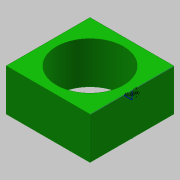
# Autodesk Inventor part: B2-Y
Saved by Autodesk Inventor 2018.1 (Build 221171000, 171)
## iProperties
Created: 2018-06-22
Part Number: B2-Y
Material: Všeobecné
Document SubType Name: Modeling
Designer: PS
Density: 1 g/cm^3
Appearance: Výchozí
Author: PS
Autodesk Inventor part; units mm, degrees
ref_plane "YZ Plane" through (0, 0, 0) normal (1, 0, 0) x (0, 1, 0)
ref_plane "XZ Plane" through (0, 0, 0) normal (0, 1, 0) x (-1, 0, 0)
sketch "Náčrt1" plane through (0, 0, 0) normal (0, 0, 1) x (1, 0, 0)
  line L0 (-500, -500) -> (500, -500)
  line L1 (500, -500) -> (500, 500)
  line L2 (500, 500) -> (-500, 500)
  line L3 (-500, 500) -> (-500, -500)
  line L4 (-500, -500) -> (500, 500) construction
  line L5 (500, -500) -> (-500, 500) construction
  circle A0 centre (0, 0) radius 400
  dimension "d0" = 1000
  dimension "d1" = 1000
  dimension "d6" = 800
  constraints: 12 end point, 2 parallel, 1 centre point, 1 coincident, 1 horizontal, 1 midpoint, 1 perpendicular
  measures "d0" distance of L1.end L0.end
  measures "d1" distance of L1.end L2.end
  measures "d6" diameter of A0
extrude "Vysunutí1" add sketch "Náčrt1" along normal blind 500
sketch "Náčrt2" plane through (500, -500, 0) normal (1, 0, 0) x (0, 0, -1)
  line L0 (-500, 0) -> (-500, 1000) projected
  line L1 (-500, 500) -> (-400, 500)
  line L2 (-400, 500) -> (-500, 400)
  point P0 (0, 500)
  dimension "d7" = 100
  dimension "d8" = 45
  constraints: 4 end point, 1 horizontal, 1 midpoint, 1 point on line
  measures "d7" distance of L1.start L1.end
  measures "d8" angle of L2 L1
ref_plane "Pracovní rovina1" through (-500, -4173.9622, 0) normal (1, 0, 0) x (0, 1, 0)
extrude "Vysunutí2" cut sketch "Náčrt2" against normal up to surface (1000 mm away)
equation "\"d1\" = d0"
